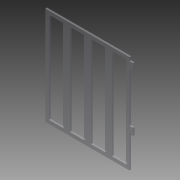
# Autodesk Inventor part: Backboard
Saved by Autodesk Inventor 2013 (Build 170138000, 138)
## iProperties
Created: 2013-01-30
Part Number: Backboard
Material: Polycarbonate, Clear
Document SubType Name: Modeling
Designer: actoennies
Mass: 39.9435 g
Surface Area: 279.838 cm^2
Volume: 33.2862 cm^3
Density: 1.2 g/cm^3
Author: actoennies
Autodesk Inventor part; units mm, degrees
ref_plane "YZ Plane" through (0, 0, 0) normal (1, 0, 0) x (0, 1, 0)
ref_plane "XZ Plane" through (0, 0, 0) normal (0, 1, 0) x (-1, 0, 0)
ref_plane "XY Plane" through (0, 0, 0) normal (0, 0, 1) x (1, 0, 0)
sketch "Sketch1" plane through (0, 0, 0) normal (0, 0, 1) x (1, 0, 0)
  line L0 (0, 0) -> (0, 177.8)
  line L1 (0, 177.8) -> (152.4, 177.8)
  line L2 (152.4, 177.8) -> (152.4, 0)
  line L3 (152.4, 0) -> (0, 0)
  dimension "d0" = 177.8
  dimension "d1" = 152.4
  constraints: 8 end point, 2 parallel, 1 perpendicular, 1 point on line, 1 vertical
  measures "d0" distance of L0.start L0.end
  measures "d1" distance of L0.end L1.end
extrude "Extrusion1" add sketch "Sketch1" along normal blind 3.175
sketch "Sketch2" plane through (0, 0, 0) normal (0, 0, -1) x (-1, 0, 0)
  line L0 (-152.4, 177.8) -> (0, 177.8) projected
  line L1 (-152.4, 0) -> (-152.4, 177.8) projected
  line L2 (0, 0) -> (-152.4, 0) projected
  line L3 (-152.4, 171.45) -> (-158.75, 171.45)
  line L4 (-158.75, 171.45) -> (-158.75, 158.75)
  line L5 (-158.75, 158.75) -> (-152.4, 158.75)
  line L6 (-152.4, 69.85) -> (-158.75, 69.85)
  line L7 (-158.75, 69.85) -> (-158.75, 57.15)
  line L8 (-158.75, 57.15) -> (-152.4, 57.15)
  dimension "d9" = 6.35
  dimension "d10" = 12.7
  dimension "d11" = 6.35
  dimension "d12" = 12.7
  dimension "d13" = 88.9
  dimension "d14" = 6.35
  constraints: 12 end point, 4 perpendicular, 4 point on line, 2 parallel
  measures "d9" distance of L3.start L3.end
  measures "d10" distance of L3.end L4.end
  measures "d11" distance of L6.start L6.end
  measures "d12" distance of L6.end L7.end
  measures "d13" distance from line of L4.end L6
  measures "d14" distance between parallel lines of L0 L3
extrude "Extrusion2" add sketch "Sketch2" against normal blind 3.175
sketch "Sketch3" plane through (0, 0, 0) normal (0, 0, -1) x (-1, 0, 0)
  line L0 (-152.4, 177.8) -> (0, 177.8) projected
  line L1 (-152.4, 171.45) -> (-152.4, 177.8) projected
  line L2 (0, 0) -> (-152.4, 0) projected
  line L3 (-146.05, 171.45) -> (-120.65, 171.45)
  line L4 (-120.65, 171.45) -> (-120.65, 6.35)
  line L5 (-120.65, 6.35) -> (-146.05, 6.35)
  line L6 (-146.05, 171.45) -> (-146.05, 6.35)
  line L7 (-107.95, 171.45) -> (-82.55, 171.45)
  line L8 (-82.55, 171.45) -> (-82.55, 6.35)
  line L9 (-82.55, 6.35) -> (-107.95, 6.35)
  line L10 (-107.95, 171.45) -> (-107.95, 6.35)
  line L11 (-69.85, 171.45) -> (-44.45, 171.45)
  line L12 (-44.45, 171.45) -> (-44.45, 6.35)
  line L13 (-44.45, 6.35) -> (-69.85, 6.35)
  line L14 (-69.85, 171.45) -> (-69.85, 6.35)
  line L15 (-31.75, 171.45) -> (-6.35, 171.45)
  line L16 (-6.35, 171.45) -> (-6.35, 6.35)
  line L17 (-6.35, 6.35) -> (-31.75, 6.35)
  line L18 (-31.75, 171.45) -> (-31.75, 6.35)
  dimension "d17" = 25.4
  dimension "d18" = 25.4
  dimension "d20" = 6.35
  dimension "d21" = 6.35
  dimension "d22" = 6.35
  dimension "d25" = 38.1
  constraints: 32 end point, 2 parallel, 1 horizontal, 1 perpendicular, 24 other
  measures "d17" distance of L3.start L3.end
  measures "d18" distance of L4.end L5.end
  measures "d20" distance between parallel lines of L0 L3
  measures "d21" distance between parallel lines of L2 L5
  measures "d22" distance from line of L1 L3.start
  measures "d25" distance of L3.end L8.start
extrude "Extrusion3" cut sketch "Sketch3" against normal blind 3.175
body "Solid1"
